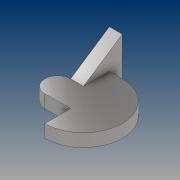
# Autodesk Inventor part: 44
Saved by Autodesk Inventor 2020.2 (Build 242310000, 310)
## iProperties
Created: 2020-09-17
Part Number: 44
Material: 鋼、碳鋼
Document SubType Name: Modeling
Designer: user
Density: 7.85 g/cm^3
Appearance: 半拋光
Mass: 217.508 g
Surface Area: 80.5878 cm^2
Volume: 27.708 cm^3
Author: user
Autodesk Inventor part; units mm, degrees
ref_plane "YZ Plane" through (0, 0, 0) normal (1, 0, 0) x (0, 1, 0)
ref_plane "XZ Plane" through (0, 0, 0) normal (0, 1, 0) x (-1, 0, 0)
ref_plane "XY Plane" through (0, 0, 0) normal (0, 0, 1) x (1, 0, 0)
sketch "草圖1" plane through (0, 0, 0) normal (0, 1, 0) x (-1, 0, 0)
  circle A0 centre (0, 0) radius 10
  line L0 (0, -10) -> (-10, -10)
  line L1 (-10, -10) -> (-10, -30)
  line L2 (-10, -30) -> (-20, -30)
  arc A1 (-20, 30) -> (-20, -30) centre (-20, 0) ccw
  line L3 (-20, 30) -> (-20, 30)
  line L4 (-20, 30) -> (-20, 10)
  line L5 (-20, 10) -> (0, 10)
  point P0 (-20, 30)
  dimension "d0" = 20
  dimension "d1" = 10
  dimension "d2" = 20
  dimension "d3" = 30
  dimension "d4" = 20
  constraints: 12 end point, 4 perpendicular, 4 point on circle, 4 tangent, 2 centre point, 1 coincident, 1 horizontal, 1 horizontal alignment, 1 parallel
  measures "d0" diameter of A0
  measures "d1" distance from line of L1 A0.centre
  measures "d2" distance of L4.end L5.end
  measures "d3" radius of A1
  measures "d4" distance of A1.centre A0.centre
extrude "擠出1" add sketch "草圖1" along normal blind 10
sketch "草圖2" plane through (10, 0, -30) normal (-1, 0, 0) x (0, 0, 1)
  line L0 (0, 0) -> (0, 10) projected
  line L1 (0, 10) -> (20, 10) projected
  line L2 (20, 0) -> (20, 10) projected
  line L3 (40, 0) -> (20, 0) projected
  line L4 (40, 10) -> (40, 0) projected
  line L5 (20, 10) -> (40, 10) projected
  line L6 (20, 0) -> (0, 0) projected
  line L7 (20, 10) -> (-10, 30)
  line L8 (-10, 30) -> (-10, 0)
  line L9 (-10, 0) -> (20, 0)
  line L10 (20, 0) -> (20, 10)
  point P0 (30, 0)
  dimension "d7" = 10
  dimension "d8" = 30
  constraints: 8 end point, 1 collinear, 1 perpendicular, 1 vertical
  measures "d7" distance between parallel lines of L8 L0
  measures "d8" distance of L7.end L8.end
extrude "擠出2" add sketch "草圖2" along normal blind 10 contours L9 L8 L7 L1 L0 | L0 L1 L2 L6
